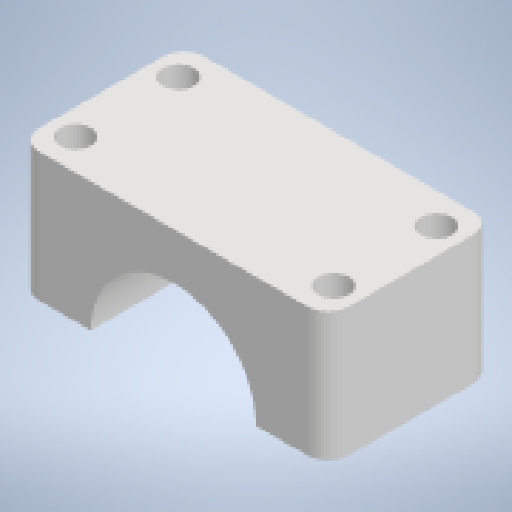
# Autodesk Inventor part: base2
Saved by Autodesk Inventor 2023 (Build 270158000, 158)
## iProperties
Created: 2022-11-13
Part Number: base2
Material: Generic
Document SubType Name: Modeling
Designer: andre
Density: 1 g/cm^3
Appearance: Default
Author: andre
Autodesk Inventor part; units mm, degrees
ref_plane "YZ Plane" through (0, 0, 0) normal (1, 0, 0) x (0, 1, 0)
ref_plane "XZ Plane" through (0, 0, 0) normal (0, 1, 0) x (-1, 0, 0)
ref_plane "XY Plane" through (0, 0, 0) normal (0, 0, 1) x (1, 0, 0)
sketch "Sketch1" plane through (0, 0, 0) normal (0, 0, 1) x (1, 0, 0)
  line L0 (0, 0) -> (30, 0)
  line L1 (30, 0) -> (30, 12.5)
  line L2 (30, 12.5) -> (0, 12.5)
  line L3 (0, 12.5) -> (0, 0)
  circle A0 centre (15, 0) radius 8
  point P0 (7, 0)
  point P1 (23, 0)
  dimension "d0" = 30
  dimension "d1" = 12.5
  dimension "d2" = 16
  constraints: 8 end point, 2 parallel, 1 centre point, 1 horizontal, 1 midpoint, 1 perpendicular
  measures "d0" distance of L2.end L1.end
  measures "d1" distance of L1.end L0.end
  measures "d2" diameter of A0
extrude "Extrusion1" add sketch "Sketch1" along normal mid plane 16 contours A0 L0 L3 L2 L1
sketch "Sketch2" plane through (0, 12.5, 8) normal (0, 1, 0) x (1, 0, 0)
  line L0 (0, 16) -> (0, 0) projected
  line L1 (30, 0) -> (0, 0) projected
  line L2 (30, 16) -> (30, 0) projected
  line L3 (0, 16) -> (30, 16) projected
  line L4 (23, 0) -> (7, 0) projected
  line L5 (15, 0) -> (15, 16)
  line L6 (0, 8) -> (30, 8)
  line L7 (2.5, 3) -> (27.5, 3)
  line L8 (27.5, 3) -> (27.5, 13)
  line L9 (27.5, 13) -> (2.5, 13)
  line L10 (2.5, 13) -> (2.5, 3)
  dimension "d5" = 25
  dimension "d6" = 10
  constraints: 12 end point, 4 coincident, 3 midpoint, 2 parallel, 1 horizontal, 1 perpendicular, 2 other
  measures "d5" distance of L9.end L8.end
  measures "d6" distance of L8.end L7.end
hole "Hole1" at (2.5, 12.5, 5) at (2.5, 12.5, -5) at (27.5, 12.5, -5) at (27.5, 12.5, 5) direction (0, -1, 0) diameter 3 end through all
fillet "Fillet1" radius 2 4 edges at (0, 6.25, 8) (30, 6.25, -8) (30, 6.25, 8) (0, 6.25, -8)
body "Solid1"
